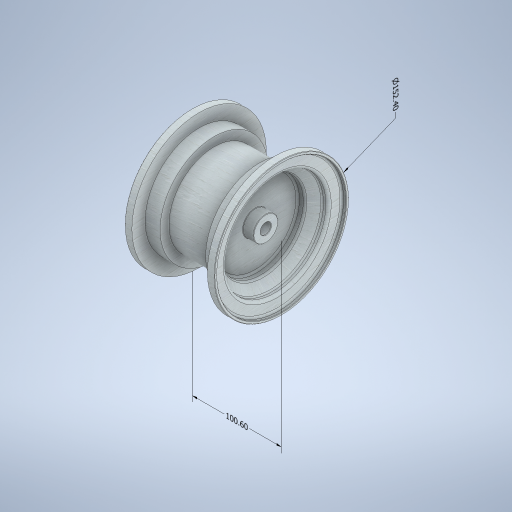
# Autodesk Inventor part: velg
Saved by Autodesk Inventor 2023 (Build 270158000, 158)
## iProperties
Created: 2023-09-02
Part Number: velg
Material: Generic
Document SubType Name: Modeling
Designer: sigit
Density: 1 g/cm^3
Appearance: Default
Author: sigit
Autodesk Inventor part; units mm, degrees
ref_plane "YZ Plane" through (0, 0, 0) normal (1, 0, 0) x (0, 1, 0)
ref_plane "XZ Plane" through (0, 0, 0) normal (0, 1, 0) x (-1, 0, 0)
ref_plane "XY Plane" through (0, 0, 0) normal (0, 0, 1) x (1, 0, 0)
sketch "Sketch1" plane through (0, 0, 0) normal (0, 0, 1) x (1, 0, 0)
  line L0 (25.8, 61.2) -> (25.8, 51.2)
  line L1 (42.8, 76.2) -> (42.8, 61.2)
  line L2 (50.8, 76.2) -> (42.8, 76.2)
  line L3 (42.8, 76.2) -> (42.8, 61.2)
  line L4 (42.8, 61.2) -> (25.8, 61.2)
  line L5 (25.8, 61.2) -> (25.8, 51.2)
  line L6 (25.8, 51.2) -> (17.8, 51.2)
  line L7 (20.8, 0) -> (20.8, 48.2)
  line L8 (20.8, 48.2) -> (28.8, 48.2)
  line L9 (28.8, 58.2) -> (28.8, 48.2)
  line L10 (45.8, 58.2) -> (28.8, 58.2)
  line L11 (45.8, 73.2) -> (45.8, 58.2)
  line L12 (50.8, 73.2) -> (45.8, 73.2)
  line L13 (50.8, 76.2) -> (50.8, 73.2)
  line L14 (0, 0) -> (93.4181, 0)
  line L15 (-25.8, 61.2) -> (-25.8, 51.2)
  line L16 (-42.8, 76.2) -> (-42.8, 61.2)
  line L17 (-50.8, 76.2) -> (-42.8, 76.2)
  line L18 (-42.8, 76.2) -> (-42.8, 61.2)
  line L19 (-42.8, 61.2) -> (-25.8, 61.2)
  line L20 (-25.8, 61.2) -> (-25.8, 51.2)
  line L21 (-25.8, 51.2) -> (-17.8, 51.2)
  line L22 (-20.8, 0) -> (-20.8, 48.2)
  line L23 (-20.8, 48.2) -> (-28.8, 48.2)
  line L24 (-28.8, 58.2) -> (-28.8, 48.2)
  line L25 (-45.8, 58.2) -> (-28.8, 58.2)
  line L26 (-45.8, 73.2) -> (-45.8, 58.2)
  line L27 (-50.8, 73.2) -> (-45.8, 73.2)
  line L28 (-50.8, 76.2) -> (-50.8, 73.2)
  line L29 (-20.8, 0) -> (20.8, 0)
  line L30 (17.8, 51.2) -> (-17.8, 51.2)
  point P0 (0, 2.9227)
  point P1 (17.8, 0)
  constraints: 62 end point, 4 parallel, 3 horizontal, 3 vertical, 2 perpendicular, 1 collinear
revolve "Revolution1" add sketch "Sketch1" angle 360 about axis through (0, 0, 0) along (1, 0, 0)
chamfer "Chamfer1" distance 10 angle 45 1 edges at (28.8, -58.2, 0)
fillet "Fillet1" radius 4 2 edges at (28.8, -48.2001, 0) (28.8, -48.2, 0)
fillet "Fillet2" radius 2 1 edges at (20.8, -48.2, 0)
fillet "Fillet3" radius 3 1 edges at (38.7999, -58.2, 0)
fillet "Fillet4" radius 3 1 edges at (45.8, -58.2, 0)
fillet "Fillet5" radius 2 1 edges at (45.8, -73.2, 0)
fillet "Fillet6" radius 0.5 4 edges at (50.8, -73.2, 0) (50.8, -76.2, 0) (-50.8, -76.2, 0) (-50.8, -73.2, 0)
fillet "Fillet7" radius 2 1 edges at (-45.8, -73.2, 0)
fillet "Fillet8" radius 3 1 edges at (-45.8, -58.2, 0)
fillet "Fillet9" radius 2 1 edges at (-20.8, -48.2, 0)
chamfer "Chamfer2" distance 10 angle 45 1 edges at (-28.8, -58.2, 0)
fillet "Fillet10" radius 2 2 edges at (-28.8, -48.2001, 0) (-28.8, -48.2, 0)
sketch "Sketch2" plane through (20.8, 0, 0) normal (1, 0, 0) x (0, 0, -1)
  circle A0 centre (0, 0) radius 14
  dimension "d34" = 28
  constraints: 1 centre point, 1 coincident
  measures "d34" diameter of A0
extrude "Extrusion1" cut sketch "Sketch2" along normal through all both and the other way through all
sketch "Sketch4" plane through (0, 0, 0) normal (1, 0, 0) x (0, 1, 0)
  circle A0 centre (0, 0) radius 6
  circle A1 centre (0, 0) radius 14
  dimension "d43" = 12
  dimension "d44" = 28
  constraints: 2 centre point, 2 coincident
  measures "d43" diameter of A0
  measures "d44" diameter of A1
extrude "Extrusion3" add sketch "Sketch4" along normal mid plane 41.6
sketch "Sketch5" plane through (-20.8, 0, 0) normal (-1, 0, 0) x (0, 0, 1)
  circle A0 centre (0, 0) radius 6 projected
  circle A1 centre (0, 0) radius 6
  circle A2 centre (0, 0) radius 14
  dimension "d47" = 12
  dimension "d48" = 28
  constraints: 2 centre point, 2 coincident
  measures "d47" diameter of A1
  measures "d48" diameter of A2
extrude "Extrusion4" add sketch "Sketch5" along normal blind 40
sketch "Sketch6" plane through (20.8, 0, 0) normal (1, 0, 0) x (0, 0, -1)
  circle A0 centre (0, 0) radius 6
  circle A1 centre (0, 0) radius 14
  dimension "d51" = 28
  constraints: 2 centre point, 2 coincident
  measures "d51" diameter of A1
extrude "Extrusion5" add sketch "Sketch6" along normal blind 12
fillet "Fillet11" radius 0.5 3 edges at (32.8, 0, 14) (32.8, 0, 6) (20.8, 0, 14)
fillet "Fillet12" radius 0.5 3 edges at (-20.8, 0, -14) (-60.8, 0, -14) (-60.8, 0, -6)
ref_plane "Work Plane1" through (-55.8, 0, 0) normal (-1, 0, 0) x (0, 0, 1)
sketch "Sketch8" plane through (-55.8, 0, 0) normal (-1, 0, 0) x (0, 0, 1)
  circle A0 centre (0, 0) radius 14
  circle A1 centre (0, 0) radius 30
  dimension "d59" = 28
  dimension "d60" = 60
  constraints: 2 centre point, 2 coincident
  measures "d59" diameter of A0
  measures "d60" diameter of A1
extrude "Extrusion6" add sketch "Sketch8" against normal blind 3
fillet "Fillet13" radius 1 2 edges at (-55.8, 0, -30) (-52.8, 0, -30)
sketch "Sketch9" plane through (-55.8, 0, 0) normal (-1, 0, 0) x (0, 0, 1)
  circle A0 centre (0, 24.25) radius 2
  circle A1 centre (-21.0011, -12.125) radius 2
  circle A2 centre (21.0011, -12.125) radius 2
  point P0 (0, 0)
  dimension "d64" = 4
  dimension "d67" = 360
  dimension "d74" = 24.25
  constraints: 3 centre point, 7 other
  measures "d64" diameter of A0
  measures "d74" distance of A0.centre point (0, 0)
extrude "Extrusion7" cut sketch "Sketch9" against normal blind 3
body "Solid1"
